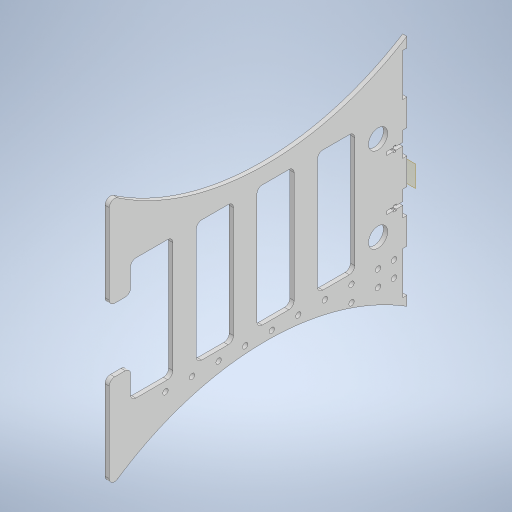
# Autodesk Inventor part: грань тела
Saved by Autodesk Inventor 2023.1 (Build 271208000, 208)
## iProperties
Created: 2024-11-21
Part Number: грань тела
Material: Типовые
Document SubType Name: Modeling
Designer: DELL
Density: 1 g/cm^3
Appearance: По умолчанию
Author: DELL
Autodesk Inventor part; units mm, degrees
ref_plane "YZ Plane" through (0, 0, 0) normal (1, 0, 0) x (0, 1, 0)
ref_plane "XZ Plane" through (0, 0, 0) normal (0, 1, 0) x (-1, 0, 0)
ref_plane "РабПлоскость1" through (0, 0, -4) normal (0, 0, 1) x (1, 0, 0)
sketch "Эскиз10" plane through (0, 0, 0) normal (1, 0, 0) x (0, 1, 0)
  line L0 (-120, -4) -> (120, -4) construction
  line L1 (120, -4) -> (120, 276) construction
  line L2 (110.389, 276) -> (-110.389, 276)
  line L3 (-120, 276) -> (-120, -4) construction
  line L4 (-110, -4) -> (110, -4)
  arc A0 (-110, -4) -> (-114.5368, 268.208) centre (-321.9309, 128.6096) ccw
  arc A1 (114.5368, 268.208) -> (110, -4) centre (321.9309, 128.6096) ccw
  arc A2 (114.5368, 268.208) -> (110.389, 276) centre (110.389, 271) ccw
  arc A3 (-110.389, 276) -> (-114.5368, 268.208) centre (-110.389, 271) ccw
  point P0 (0, 0)
  point P1 (0, -4)
  dimension "d50" = 240
  dimension "d51" = 280
  dimension "d52" = 220
  dimension "d53" = 250
  dimension "d54" = 250
  dimension "d55" = 5
  constraints: 10 end point, 10 point on circle, 4 centre point, 4 tangent, 2 horizontal, 2 midpoint, 2 parallel, 2 point on line, 1 equal radius, 1 perpendicular
  measures "d50" distance of L3.start L1.end
  measures "d51" distance of L1.end L0.end
  measures "d52" distance of L4.start L4.end
  measures "d53" radius of A0
  measures "d54" radius of A1
  measures "d55" radius of A2
extrude "Выдавливание6" add sketch "Эскиз10" along normal mid plane 4
sketch "Эскиз12" plane through (2, 0, 0) normal (1, 0, 0) x (0, 0, -1)
  line L0 (4.1067, -100.9593) -> (0, -100.9593)
  line L1 (0, -100.9593) -> (0, -60.9593)
  line L2 (0, -60.9593) -> (4, -60.9593)
  line L3 (4, 110) -> (4, -110) projected
  line L4 (4, -110) -> (4, 110) projected
  line L5 (4, -35.9593) -> (0, -35.9593)
  line L6 (0, -35.9593) -> (0, -12.5)
  line L7 (0, -12.5) -> (4, -12.5)
  line L8 (4, 12.5) -> (0, 12.5)
  line L9 (0, 12.5) -> (0, 35.5004)
  line L10 (0, 35.5004) -> (4, 35.5004)
  line L11 (4, 60.5004) -> (0, 60.5004)
  line L12 (0, 60.5004) -> (0, 100.5004)
  line L13 (0, 100.5004) -> (4, 100.5004)
  point P0 (0, 0)
  point P1 (4, 12.5)
  point P2 (4, 35.5004)
  point P3 (4, -35.9593)
  point P4 (4, -12.5)
  point P5 (4, -100.9593)
  constraints: 24 end point, 10 perpendicular, 7 point on line, 2 horizontal, 8 other
extrude "Выдавливание7" cut sketch "Эскиз12" against normal blind 4
sketch "Эскиз13" plane through (2, 0, 0) normal (1, 0, 0) x (0, 0, -1)
  line L0 (-15, -22.6546) -> (-15, -25.8046)
  line L1 (0, -25.7683) -> (0, -22.691)
  line L2 (0, -35.9593) -> (0, -12.5) projected
  line L3 (-6.1608, -27.016) -> (-8.4608, -27.016)
  line L4 (-8.4608, -21.516) -> (-6.1608, -21.516)
  line L5 (-15, -24.2296) -> (0, -24.2296) construction
  line L6 (0, -12.5) -> (0, -35.9593) projected
  line L7 (-8.4608, -27.016) -> (-8.4608, -25.8046)
  line L8 (-8.4608, -22.6546) -> (-8.4608, -21.516)
  line L9 (-15, -25.8046) -> (-8.4608, -25.8046)
  line L10 (-6.1608, -25.7683) -> (0, -25.7683)
  line L11 (-6.1608, -21.516) -> (-6.1608, -22.691)
  line L12 (-6.1608, -25.7683) -> (-6.1608, -27.016)
  line L13 (0, -22.691) -> (-6.1608, -22.691)
  line L14 (-8.4608, -22.6546) -> (-15, -22.6546)
  line L15 (0, 12.5) -> (0, 35.5004) projected
  line L16 (0, 18.7449) -> (0, 30.6124)
  line L17 (0, 22.4252) -> (0, 25.5752)
  line L18 (-15, 25.5752) -> (-15, 22.4252)
  line L19 (-8.65, 21.2502) -> (-6.35, 21.2502)
  line L20 (-6.35, 26.7502) -> (-8.65, 26.7502)
  line L21 (-15, 24.0002) -> (0, 24.0002) construction
  line L22 (-8.65, 26.7502) -> (-8.65, 25.5752)
  line L23 (-8.65, 22.4252) -> (-8.65, 21.2502)
  line L24 (-15, 22.4252) -> (-8.65, 22.4252)
  line L25 (-6.35, 22.4252) -> (0, 22.4252)
  line L26 (-6.35, 21.2502) -> (-6.35, 22.4252)
  line L27 (-6.35, 25.5752) -> (-6.35, 26.7502)
  line L28 (0, 25.5752) -> (-6.35, 25.5752)
  line L29 (-8.65, 25.5752) -> (-15, 25.5752)
  circle A0 centre (-23.1563, -40) radius 9
  line L30 (4, -35.9593) -> (4, -60.9593) projected
  line L31 (4, 35.5004) -> (4, 60.5004) projected
  line L32 (0, 0) -> (-64.5188, 0) construction
  circle A1 centre (-23.1563, 40) radius 9
  dimension "d60" = 15
  dimension "d61" = 3.15
  dimension "d62" = 2.3
  dimension "d63" = 5.5
  dimension "d64" = 6.35
  dimension "d70" = 15
  dimension "d71" = 3.15
  dimension "d72" = 2.3
  dimension "d73" = 5.5
  dimension "d77" = 18
  dimension "d114" = 80
  constraints: 56 end point, 20 parallel, 10 perpendicular, 8 midpoint, 7 horizontal, 2 centre point, 2 point on line, 1 symmetric about line, 1 other
  measures "d60" distance of L1.start L0.end
  measures "d61" distance of L0.end L0.start
  measures "d62" distance of L4.start L4.end
  measures "d63" distance of L3.end L4.start
  measures "d64" distance of point (0, -24.23) L11.end
  measures "d70" distance of L18.start L17.end
  measures "d71" distance of L17.end L17.start
  measures "d72" distance of L20.end L20.start
  measures "d73" distance of L20.start L19.end
  measures "d77" diameter of A0
  measures "d114" distance of A1.centre A0.centre
extrude "Выдавливание8" cut sketch "Эскиз13" against normal blind 4
sketch "Эскиз15" plane through (-2, 0, 0) normal (-1, 0, 0) x (0, 0, 1)
  line L0 (0, 75.3813) -> (0, -75.381) construction
  line L1 (0, 57.0002) -> (0, 61.0002) construction
  line L2 (0, 61.0002) -> (276, 61.0002) construction
  line L3 (276, 61.0002) -> (276, 57.0002) construction
  line L4 (276, 57.0002) -> (0, 57.0002) construction
  line L5 (0, -61.2296) -> (0, -57.2296) construction
  line L6 (0, -57.2296) -> (276, -57.2296) construction
  line L7 (276, -57.2296) -> (276, -61.2296) construction
  line L8 (276, -61.2296) -> (0, -61.2296) construction
  circle A0 centre (23.1563, 40) radius 9 construction
  circle A1 centre (23.1563, -40) radius 9 construction
  line L9 (45.1563, 57.0002) -> (45.1563, -52.2296) construction
  line L10 (107.1563, 57.0002) -> (132.1563, 57.0002)
  line L11 (137.1563, 52.0002) -> (137.1563, -52.2296)
  line L12 (132.1563, -57.2296) -> (107.1563, -57.2296)
  line L13 (102.1563, -52.2296) -> (102.1563, 52.0002)
  line L14 (221.1563, 57.0002) -> (251, 57.0002)
  line L15 (251, -57.2296) -> (221.1563, -57.2296)
  line L16 (216.1563, -52.2296) -> (216.1563, 52.0002)
  line L17 (276, 35.0002) -> (276, 110.389)
  line L18 (164.1563, 57.0002) -> (189.1563, 57.0002)
  line L19 (194.1563, 52.0002) -> (194.1563, -52.2296)
  line L20 (189.1563, -57.2296) -> (164.1563, -57.2296)
  line L21 (159.1563, -52.2296) -> (159.1563, 52.0002)
  line L22 (50.1563, 57.0002) -> (75.1563, 57.0002)
  line L23 (80.1563, 52.0002) -> (80.1563, -52.2296)
  line L24 (75.1563, -57.2296) -> (50.1563, -57.2296)
  line L25 (45.1563, -57.2296) -> (45.1563, 52.0002)
  arc A2 (50.1563, 57.0002) -> (45.1563, 52.0002) centre (50.1563, 52.0002) ccw
  arc A3 (80.1563, 52.0002) -> (75.1563, 57.0002) centre (75.1563, 52.0002) ccw
  arc A4 (45.1563, -52.2296) -> (50.1563, -57.2296) centre (50.1563, -52.2296) ccw
  arc A5 (75.1563, -57.2296) -> (80.1563, -52.2296) centre (75.1563, -52.2296) ccw
  arc A6 (107.1563, 57.0002) -> (102.1563, 52.0002) centre (107.1563, 52.0002) ccw
  arc A7 (137.1563, 52.0002) -> (132.1563, 57.0002) centre (132.1563, 52.0002) ccw
  arc A8 (102.1563, -52.2296) -> (107.1563, -57.2296) centre (107.1563, -52.2296) ccw
  arc A9 (132.1563, -57.2296) -> (137.1563, -52.2296) centre (132.1563, -52.2296) ccw
  arc A10 (164.1563, 57.0002) -> (159.1563, 52.0002) centre (164.1563, 52.0002) ccw
  arc A11 (194.1563, 52.0002) -> (189.1563, 57.0002) centre (189.1563, 52.0002) ccw
  arc A12 (189.1563, -57.2296) -> (194.1563, -52.2296) centre (189.1563, -52.2296) ccw
  arc A13 (159.1563, -52.2296) -> (164.1563, -57.2296) centre (164.1563, -52.2296) ccw
  arc A14 (221.1563, 57.0002) -> (216.1563, 52.0002) centre (221.1563, 52.0002) ccw
  arc A15 (256, 52.0002) -> (251, 57.0002) centre (251, 52.0002) ccw
  arc A16 (251, -57.2296) -> (256, -52.2296) centre (251, -52.2296) ccw
  arc A17 (216.1563, -52.2296) -> (221.1563, -57.2296) centre (221.1563, -52.2296) ccw
  line L26 (271, -29.9962) -> (261, -29.9962)
  line L27 (261, 30.0002) -> (271, 30.0002)
  line L28 (276, -13.2762) -> (255.9998, 30.0002) construction
  line L29 (256.0015, -29.9962) -> (276, 13.2766) construction
  line L30 (276, 41.3488) -> (276, 1056.4994)
  line L31 (276, 110.389) -> (276, -110.389) projected
  arc A18 (271, 30.0002) -> (276, 35.0002) centre (271, 35.0002) ccw
  line L32 (276, -34.9962) -> (276, -49)
  arc A19 (276, -34.9962) -> (271, -29.9962) centre (271, -34.9962) ccw
  line L33 (276, 57.0002) -> (276, -57.2296)
  line L34 (256, 52.0002) -> (256, 35.0002)
  line L35 (256, -34.9962) -> (256, -52.2296)
  arc A20 (256, 35.0002) -> (261, 30.0002) centre (261, 35.0002) ccw
  arc A21 (261, -29.9962) -> (256, -34.9962) centre (261, -34.9962) ccw
  point P0 (45.1563, -57.2296)
  point P1 (102.1563, 57.0002)
  point P2 (137.1563, -57.2296)
  point P3 (216.1563, 57.0002)
  point P4 (256, -57.2296)
  point P5 (166, -0.1147)
  point P6 (159.1563, 57.0002)
  point P7 (194.1563, -57.2296)
  point P8 (80.1563, -57.2296)
  point P9 (50.1563, -52.2296)
  point P10 (269.8643, 0.0002)
  point P11 (276, 30.0002)
  point P12 (276, -29.9962)
  point P13 (256, 29.9998)
  point P14 (256, -29.9994)
  point P15 (276, -34.9998)
  point P16 (276, 35.0002)
  point P17 (45.1563, -52.2296)
  dimension "d99" = 22
  dimension "d101" = 35
  dimension "d107" = 35
  dimension "d108" = 22
  dimension "d109" = 22
  dimension "d110" = 35
  dimension "d111" = 5
  dimension "d117" = 5
  dimension "d118" = 5
  dimension "d119" = 5
  dimension "d140" = 22
  constraints: 68 end point, 41 tangent, 40 point on circle, 37 point on line, 20 centre point, 16 equal radius, 10 parallel, 6 perpendicular, 5 horizontal, 28 other
  measures "d99" distance from line of A0.centre L9
  measures "d101" distance between parallel lines of L11 L13
  measures "d107" distance between parallel lines of L21 L19
  measures "d108" distance between parallel lines of L16 L19
  measures "d109" distance between parallel lines of L21 L11
  measures "d110" distance from line of L25.start L23
  measures "d111" radius of A2
  measures "d117" radius of A18
  measures "d118" radius of A19
  measures "d119" radius of A20
  measures "d140" distance between parallel lines of L23 L13
extrude "Выдавливание10" cut sketch "Эскиз15" against normal blind 10
sketch "Эскиз17" plane through (-2, 0, 0) normal (-1, 0, 0) x (0, 0, 1)
  circle A0 centre (23.1563, -40) radius 9 projected
  circle A1 centre (23.1563, -66) radius 2.5
  line L0 (23.1563, -66) -> (240.0521, -66) construction
  circle A2 centre (48.1563, -66) radius 2.5
  circle A3 centre (73.1563, -66) radius 2.5
  circle A4 centre (98.1563, -66) radius 2.5
  circle A5 centre (123.1563, -66) radius 2.5
  circle A6 centre (148.1563, -66) radius 2.5
  circle A7 centre (173.1563, -66) radius 2.5
  circle A8 centre (198.1563, -66) radius 2.5
  circle A9 centre (223.1563, -66) radius 2.5
  circle A10 centre (248.1563, -66) radius 2.5
  circle A11 centre (48.1563, -81) radius 2.5
  circle A12 centre (8.1563, -66) radius 2.5
  circle A13 centre (23.1563, -81) radius 2.5
  circle A14 centre (8.1563, -81) radius 2.5
  point P0 (0, 0)
  dimension "d120" = 5
  dimension "d123" = 25
  dimension "d128" = 26
  dimension "d132" = 5
  dimension "d134" = 15
  dimension "d135" = 5
  dimension "d136" = 15
  dimension "d137" = 5
  constraints: 14 centre point, 2 end point, 2 horizontal, 18 other
  measures "d120" diameter of A1
  measures "d123" distance of L0.start A2.centre
  measures "d128" distance of A0.centre L0.start
  measures "d132" diameter of A11
  measures "d134" distance of A11.centre A2.centre
  measures "d135" diameter of A12
  measures "d136" distance of L0.start A12.centre
  measures "d137" diameter of A13
extrude "Выдавливание11" cut sketch "Эскиз17" against normal blind 10 contours A1 | A2 | A3 | A4 | A5 | A6 | A7 | A8 | A9 | A11 | A12 | A13 | A14
